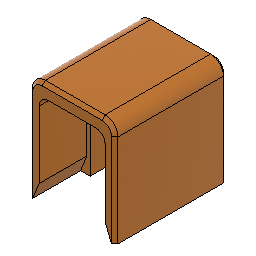
Krytka žebříku v5 (Autodesk Fusion 360 design; units mm, degrees)
Autodesk Fusion 360 part; units mm, degrees
sketch "Sketch1" plane through (0, 0, 0) normal (0, 0, 1) x (1, 0, 0)
  line L0 (-9.35, 0) -> (-9.35, 29)
  line L1 (-10.35, 29) -> (0, 29)
  line L2 (0, 33) -> (-13.35, 33)
  line L3 (-13.35, 33) -> (-13.35, 0)
  line L4 (-13.35, 0) -> (-9.35, 0)
  line L5 (-10.35, 0) -> (-10.35, 29)
  line L6 (0, 2.5) -> (0, 20)
  line L7 (13.35, 0) -> (9.35, 0)
  line L8 (0, 33) -> (13.35, 33)
  line L9 (13.35, 33) -> (13.35, 0)
  line L10 (10.35, 0) -> (10.35, 29)
  line L11 (10.35, 29) -> (0, 29)
  line L12 (9.35, 0) -> (9.35, 29)
  line L13 (5.5, 29.5) -> (-5.5, 29.5)
  line L14 (-5.5, 29.5) -> (-5.5, 28.5)
  line L15 (-5.5, 28.5) -> (5.5, 28.5)
  line L16 (5.5, 28.5) -> (5.5, 29.5)
  line L17 (5.5, 29.5) -> (-5.5, 28.5) construction
  line L18 (-5.5, 29.5) -> (5.5, 28.5) construction
  point P0 (0, 29)
  dimension "d1" = 9.35
  dimension "d3" = 4
  dimension "d4" = 4
  dimension "d5" = 29
  dimension "d18" = 1
  dimension "d19" = 11
  dimension "d20" = 1
  constraint vertical L0
  constraint perpendicular L0 L1
  constraint horizontal L2
  constraint perpendicular L2 L3
  constraint perpendicular L0 L4
  constraint vertical origin L1.end
  constraint vertical origin L2.start
  constraint horizontal origin L0.start
  constraint symmetric L0.start L6 L7.end
  constraint symmetric L0.end L6 L12.end
  constraint symmetric P0 L6 L1.end
  constraint symmetric L2.start L6 L8.start
  constraint symmetric L2.end L6 L8.end
  constraint symmetric L3.end L6 L7.start
  constraint symmetric L5.start L6 L10.start
  constraint symmetric L1.start L6 L10.end
  constraint coincident L5 L1.start
  constraint parallel L0 L5
  constraint coincident L0.end L1
  constraint coincident L10 L11.start
  constraint coincident L12.end L11
  constraint coincident L1.start L5.end
  constraint horizontal L5.start origin
  constraint horizontal L13
  constraint perpendicular L13 L14
  constraint parallel L13 L15
  constraint parallel L14 L16
  constraint coincident L17 P0
  constraint coincident L18 P0
  constraint coincident P0 L1.end
  measures "d1" distance of L0.end P0
  measures "d3" distance of L0.start L3.end
  measures "d4" distance of L1 L2
  measures "d5" distance of L0.start L0.end
  measures "d18" distance of L0.start L5.start
  measures "d19" distance of L14.end L15.end
  measures "d20" distance of L13.end L14.end
extrude "Extrude1" add sketch "Sketch1" against normal blind 20 contours L0 L1 L4 L5 | L1 L2 L3 L4 L5 L7 L8 L9 L10 L11 L13 L14 L16 | L7 L10 L11 L12
extrude "Extrude2" add sketch "Sketch1" along normal blind 15 contours L1 L2 L3 L4 L5 L7 L8 L9 L10 L11 L13 L14 L16 | L1 L11 L13 L14 L16
chamfer "Chamfer1" distance 2 distance2 5 1 edges at (-10.35, 0, 7.5) measured on face at (-11.0167, 0, -13.3333)
chamfer "Chamfer1" distance 5 distance2 2 1 edges at (10.35, 0, 7.5) measured on face at (10.35, 9.6667, 5)
fillet "Fillet1" radius 4 2 edges at (-13.35, 33, -2.5) (13.35, 33, -2.5)
fillet "Fillet2" radius 3 4 edges at (-9.35, 29, -10) (-10.35, 29, 7.5) (9.35, 29, -10) (10.35, 29, 7.5)
chamfer "Chamfer3" distance 1 angle 45 10 edges at (-13.35, 14.5, -20) (-12.1784, 31.8284, -20) (0, 33, -20) (12.1784, 31.8284, -20) (13.35, 14.5, -20) (-13.35, 14.5, 15) (13.35, 14.5, 15) (12.1784, 31.8284, 15) (0, 33, 15) (-12.1784, 31.8284, 15)
equation "d1 = ( 18.7 / 2 ) * 1 mm"
equation "w = 4 mm"
named bodies: "Kryt žebříku"
